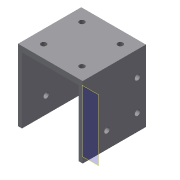
# Autodesk Inventor part: Assembly_Cube_Laser_Multicolour_insert_v3
Saved by Autodesk Inventor 2022 (Build 260153000, 153)
## iProperties
Created: 2021-12-20
Part Number: Assembly_Cube_Laser_Multicolour_insert_v3
Material: Generisch
Document SubType Name: Modeling
Designer: diederichbenedict
Density: 1 g/cm^3
Appearance: Vorgabe
Author: diederichbenedict
Autodesk Inventor part; units mm, degrees
ref_plane "YZ Plane" through (0, 0, 0) normal (1, 0, 0) x (0, 1, 0)
ref_plane "XZ Plane" through (0, 0, 0) normal (0, 1, 0) x (-1, 0, 0)
ref_plane "Arbeitsebene1" through (49.7, 8, -8.38) normal (0, 0, -1) x (-1, 0, 0)
sketch "Skizze1" plane through (49.7, 8, -8.38) normal (0, 0, -1) x (-1, 0, 0)
  line L0 (2, 0) -> (2, 41.6) projected
  line L1 (7.88, 0) -> (2, 0) projected
  line L2 (7.88, 34.1) -> (7.88, 0) projected
  line L3 (47.7, 34.1) -> (7.88, 34.1) projected
  line L4 (47.7, 41.6) -> (47.7, 34.1) projected
  line L5 (2, 41.6) -> (47.7, 41.6) projected
  line L6 (40.85, 0) -> (40.85, -4.62) projected
  line L7 (40.85, -4.62) -> (8.85, -4.62) projected
  line L8 (8.85, -4.62) -> (8.85, 0) projected
  line L9 (2, 0) -> (8.85, 0) projected
  line L10 (2, -7.5) -> (2, 0) projected
  line L11 (47.7, -7.5) -> (2, -7.5) projected
  line L12 (47.7, 34.1) -> (47.7, -7.5) projected
  line L13 (41.82, 34.1) -> (47.7, 34.1) projected
  line L14 (41.82, 0) -> (41.82, 34.1) projected
  line L15 (40.85, 0) -> (41.82, 0) projected
  line L16 (10.35, -3.12) -> (10.35, 34.38) projected
  line L17 (39.35, 34.38) -> (39.35, -3.12) projected
  line L18 (39.35, 34.38) -> (39.35, -3.12) projected
  line L19 (39.35, 34.38) -> (10.35, 34.38) projected
  line L20 (10.35, -3.12) -> (10.35, 34.38) projected
  line L21 (39.35, -3.12) -> (10.35, -3.12) projected
  line L22 (10.35, -3.12) -> (39.35, -3.12) construction
  line L23 (39.35, -3.12) -> (39.35, 34.38) construction
  line L24 (39.35, 34.38) -> (10.35, 34.38) construction
  line L25 (10.35, 34.38) -> (10.35, -3.12) construction
  line L26 (10.05, 34.68) -> (39.65, 34.68) construction
  line L27 (39.65, 34.68) -> (39.65, -3.42) construction
  line L28 (39.65, -3.42) -> (10.05, -3.42) construction
  line L29 (10.05, -3.42) -> (10.05, 34.68) construction
  line L30 (10.05, 0.3432) -> (7.98, 0.3432)
  line L31 (7.98, 0.3432) -> (7.98, 37.6)
  line L32 (7.98, 37.6) -> (10.05, 37.6)
  line L33 (10.05, 37.6) -> (10.05, 0.3432)
  line L34 (10.05, 37.6) -> (24.85, 37.6)
  line L35 (24.85, 37.6) -> (24.85, 34.68)
  line L36 (24.85, 34.68) -> (10.05, 34.68)
  line L37 (10.05, 34.68) -> (10.05, 37.6)
  point P0 (49.7, -8)
  point P1 (24.85, 34.68)
  dimension "d1" = 0.3
  dimension "d2" = 0.1
  dimension "d3" = 4
  constraints: 32 end point, 8 parallel, 4 perpendicular, 3 horizontal, 2 point on line, 1 midpoint, 3 other
  measures "d1" distance between parallel lines of L24 L26
  measures "d2" distance between parallel lines of L31 L2
  measures "d3" distance between parallel lines of L5 L34
ref_plane "Arbeitsebene2" through (41.82, 8, -41.82) normal (0, 0, 1) x (1, 0, 0)
extrude "Extrusion1" add sketch "Skizze1" along normal blind 33 contours L31 L32 L33 L3 | L3 L33 L30 L31 | L33 L34 L35 L36
sketch "Skizze2" plane through (41.72, 8.3432, -8.38) normal (1, 0, 0) x (0, 0, -1)
  circle A0 centre (12.6606, 8.6268) radius 1.4 projected
  circle A1 centre (28.5855, 24.6268) radius 1.4 projected
  circle A2 centre (28.5855, 8.6268) radius 1.4 projected
  point P0 (-8.38, -8.3432)
extrude "Extrusion2" cut sketch "Skizze2" against normal blind 33
sketch "Skizze3" plane through (24.85, 45.6, -8.38) normal (0, 1, 0) x (1, 0, 0)
  line L0 (0, 0) -> (16.87, 0) projected
  line L1 (16.87, 0) -> (16.87, 33) projected
  line L2 (0, 33) -> (16.87, 33) projected
  line L3 (0, 0) -> (0, 33) projected
  line L4 (-10, 6.5) -> (10, 6.5)
  line L5 (10, 6.5) -> (10, 26.5)
  line L6 (10, 26.5) -> (-10, 26.5)
  line L7 (-10, 26.5) -> (-10, 6.5)
  line L8 (-10, 6.5) -> (10, 26.5) construction
  line L9 (10, 6.5) -> (-10, 26.5) construction
  circle A0 centre (10, 26.5) radius 1.4
  circle A1 centre (10, 6.5) radius 1.4
  point P0 (-24.85, -8.38)
  point P1 (0, 16.5)
  dimension "d8" = 20
  dimension "d9" = 20
  dimension "d10" = 2.8
  dimension "d11" = 2.8
  constraints: 12 end point, 3 midpoint, 2 centre point, 2 coincident, 2 parallel, 1 horizontal, 1 perpendicular
  measures "d8" distance of L6.end L5.end
  measures "d9" distance of L5.end L4.end
  measures "d10" diameter of A0
  measures "d11" diameter of A1
extrude "Extrusion3" cut sketch "Skizze3" against normal blind 33 contours A1 L5 L4 | L4 L5 A1 | A0 L5 L6 | L6 L5 A0
mirror "Spiegeln1" about plane through (24.85, 42.68, -8.38) normal (-1, 0, 0) of "Extrusion1", "Extrusion2", "Extrusion3"
